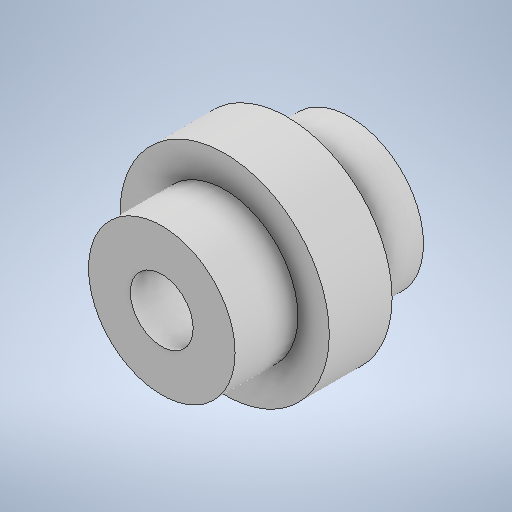
# Autodesk Inventor part: 26a
Saved by Autodesk Inventor 2025.1 (Build 291241000, 241)
## iProperties
Created: 2024-09-13
Part Number: 26a
Material: Generisch
Document SubType Name: Modeling
Designer: ffogue
Density: 1 g/cm^3
Appearance: Vorgabe
Author: ffogue
Autodesk Inventor part; units mm, degrees
ref_plane "YZ Plane" through (0, 0, 0) normal (1, 0, 0) x (0, 1, 0)
ref_plane "XZ Plane" through (0, 0, 0) normal (0, 1, 0) x (-1, 0, 0)
ref_plane "XY Plane" through (0, 0, 0) normal (0, 0, 1) x (1, 0, 0)
sketch "Sketch1" plane through (0, 0, 0) normal (0, 0, 1) x (1, 0, 0)
  line L0 (0, 9) -> (3.5, 9)
  line L1 (3.5, 9) -> (3.5, 6)
  line L2 (3.5, 6) -> (5, 6)
  line L3 (5, 6) -> (5, 3)
  line L4 (5, 3) -> (3.5, 3)
  line L5 (3.5, 3) -> (3.5, 0)
  line L6 (3.5, 0) -> (0, 0)
  line L7 (0, 0) -> (0, 9)
  dimension "d0" = 3
  dimension "d1" = 3
  dimension "d2" = 3
  dimension "d3" = 7
  dimension "d4" = 10
  constraints: 16 end point, 5 perpendicular, 2 point on line, 1 coincident, 1 horizontal, 1 vertical
  measures "d0" distance of L0.end L1.end
  measures "d1" distance of L2.end L3.end
  measures "d2" distance of L4.end L5.end
  measures "d3" diameter of L1 L7
  measures "d4" diameter of L3 L7
revolve "Revolution1" add sketch "Sketch1" angle 360 about axis through (0, 0, 0) along (0, 1, 0)
sketch "Sketch2" plane through (0, 9, 0) normal (0, 1, 0) x (1, 0, 0)
  circle A0 centre (0, 0) radius 3.5 projected
  constraints: 1 coincident
hole "Hole1" at (0, 9, 0) direction (0, -1, 0) diameter 3 depth 9 countersink diameter 6 countersink angle 90
body "Solid1"
